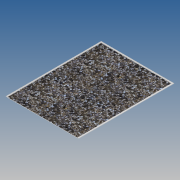
# Autodesk Inventor part: Parkeervak
Saved by Autodesk Inventor 2020 (Build 240168000, 168)
## iProperties
Created: 2019-11-19
Part Number: Parkeervak
Material: Generic
Document SubType Name: Modeling
Designer: Berkant
Density: 1 g/cm^3
Appearance: Default
Author: Berkant
Autodesk Inventor part; units mm, degrees
ref_plane "YZ Plane" through (0, 0, 0) normal (1, 0, 0) x (0, 1, 0)
ref_plane "XZ Plane" through (0, 0, 0) normal (0, 1, 0) x (-1, 0, 0)
ref_plane "XY Plane" through (0, 0, 0) normal (0, 0, 1) x (1, 0, 0)
sketch "Sketch1" plane through (0, 0, 0) normal (0, 1, 0) x (-1, 0, 0)
  line L0 (0, 0) -> (-300, 0)
  line L1 (-300, 0) -> (-300, -400)
  line L2 (-300, -400) -> (0, -400)
  line L3 (0, -400) -> (0, 0)
  dimension "d0" = 300
  dimension "d1" = 400
  constraints: 8 end point, 2 parallel, 1 horizontal, 1 perpendicular
  measures "d0" distance of L2.end L1.end
  measures "d1" distance of L1.end L0.end
extrude "Extrusion1" add sketch "Sketch1" along normal blind 1
sketch "Sketch2" plane through (0, 1, 0) normal (0, 1, 0) x (1, 0, 0)
  line L0 (0, 0) -> (300, 0) projected
  line L1 (0, 0) -> (-5, 0)
  line L2 (-5, 0) -> (-5, 405)
  line L3 (-5, 405) -> (0, 405)
  line L4 (0, 405) -> (0, 0)
  line L5 (300, 0) -> (305, 0)
  line L6 (305, 0) -> (305, 405)
  line L7 (305, 405) -> (300, 405)
  line L8 (300, 405) -> (300, 0)
  line L9 (0, 400) -> (0, 0) projected
  line L10 (300, 405) -> (0, 405)
  line L11 (0, 405) -> (0, 400)
  line L12 (0, 400) -> (300, 400)
  line L13 (300, 400) -> (300, 405)
  dimension "d4" = 5
  dimension "d5" = 405
  dimension "d6" = 5
  dimension "d7" = 405
  constraints: 24 end point, 6 parallel, 3 horizontal, 3 perpendicular
  measures "d4" distance of L2.end L3.end
  measures "d5" distance of L1.end L2.end
  measures "d6" distance of L7.end L6.end
  measures "d7" distance of L6.end L5.end
extrude "Extrusion2" add sketch "Sketch2" along normal blind 1 contours L1 L2 L3 L4 | L8 L7 L6 L5 | L4 L10 L8 L12
body "Solid1"
